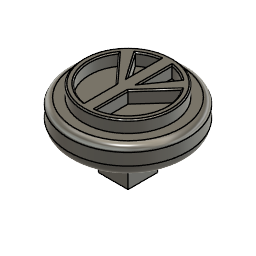
PIN2 (Autodesk Fusion 360 design; units mm, degrees)
Autodesk Fusion 360 part; units mm, degrees
sketch "Sketch2" plane through (0, 6, 0) normal (0, 1, 0) x (-1, 0, 0)
  line L0 (0, -10) -> (0, 0)
  line L1 (0, 0) -> (-5, 0)
  line L2 (-5, 0) -> (-5, -10)
  line L3 (-5, -10) -> (0, -10)
  line L4 (-5, -7.5) -> (0, -7.5)
  line L5 (0, -7.5) -> (0, -2.5)
  line L6 (0, -2.5) -> (-5, -2.5)
  line L7 (-5, -2.5) -> (-5, -7.5)
  dimension "d39" = 5
  dimension "d40" = 5
  dimension "d41" = 2.5
  constraint horizontal L4
  constraint vertical L5
  constraint horizontal L6
  constraint vertical L7
  constraint collinear L2 L7
  measures "d39" distance of L4.start L4.end
  measures "d40" distance of L4.start L6.end
  measures "d41" distance of L3 L4
extrude "Extrude2" add sketch "Sketch2" along normal blind 6 contours L0 L2 L4 L5 L6 L7 makes body 1
sketch "Sketch3" plane through (0, 12, 0) normal (0, 1, 0) x (-1, 0, 0)
  circle A0 centre (-2.5, -5) radius 10
  line L0 (-5, -2.5) -> (-5, -7.5)
  line L1 (-5, -7.5) -> (0, -7.5)
  line L2 (0, -7.5) -> (0, -2.5)
  line L3 (0, -2.5) -> (-5, -2.5)
  dimension "d12" = 20
  measures "d12" diameter of A0
extrude "Extrude3" add sketch "Sketch3" along normal blind 5 contours A0 | L0 L1 L2 L3 makes body 2
fillet "Fillet1" radius 1 1 edges at (11.8233, 17, -8.6162) on bodies 2
fillet "Fillet2" radius 2 1 edges at (11.8233, 12, -8.6162) on bodies 2
sketch "Sketch4" plane through (0, 17, 0) normal (0, 1, 0) x (-1, 0, 0)
  circle A0 centre (-2.5, -5) radius 9
  circle A1 centre (-2.5, -5) radius 6.5
  circle A2 centre (-2.5, -5) radius 7.5
  line L0 (-3.5, -11.4226) -> (-3.5, 1.4226)
  line L1 (-1.5, -11.4226) -> (-1.5, 1.4226)
  line L2 (-1.5, -4) -> (2.8204, -8.7341)
  line L3 (1.4333, -10.1749) -> (-1.5, -6)
  line L4 (-2.5, 1.5) -> (-2.5, -11.5)
  line L5 (-3.5, -4) -> (-7.8204, -8.7341)
  line L6 (-6.4333, -10.1749) -> (-3.5, -6)
  point P0 (-1.5, -11.4226)
  point P1 (-3.5, -11.4226)
  point P2 (-2.5, -11.5)
  point P3 (-1.5, -5)
  point P4 (2.1847, -9.506)
  dimension "d21" = 13
  dimension "d22" = 15
  dimension "d23" = 2
  dimension "d24" = 1
  dimension "d25" = 2
  dimension "d27" = 1
  dimension "d28" = 1
  dimension "d29" = 2
  constraint concentric A0 A1
  constraint concentric A1 A2
  constraint coincident A1 P0
  constraint coincident A1 P1
  constraint coincident A1 P2
  constraint vertical A0.centre L4.end
  constraint coincident P1 L0.start
  constraint coincident A1 L0.end
  constraint vertical L0
  constraint coincident P0 L1.start
  constraint coincident A1 L1.end
  constraint parallel L0 L1
  constraint coincident L1 L2.start
  constraint coincident A1 L2.end
  constraint coincident A1 L3.start
  constraint coincident L1 L3.end
  constraint midpoint L1 P3
  constraint coincident A1 P4
  constraint coincident A1 L4.start
  constraint coincident P2 L4.end
  constraint vertical L4
  constraint symmetric L2.start L4 L5.start
  constraint symmetric L2.end L4 L5.end
  constraint symmetric L3.start L4 L6.start
  constraint symmetric L3.end L4 L6.end
  measures "d21" diameter of A1
  measures "d22" diameter of A2
  measures "d23" distance of P0 P1
  measures "d24" horizontal distance of P0 P2
  measures "d25" distance of L2.end L3.start
  measures "d27" distance of L2.start P3
  measures "d28" distance of L2.end P4
  measures "d29" distance of L2.start L3.end
extrude "Extrude4" add sketch "Sketch4" along normal blind 2 contours A1 L1 L4 | A1 L1 L2 L3 | A1 L0 L4 | A1 L0 L5 L6 | A2 bodies 2
fillet "Fillet3" radius 0.2 13 edges at (4.9666, 19, -8.0874) (5.0443, 19, -10.9813) (3.5, 19, -8.7113) (9.4925, 19, -7.7121) (5.6602, 19, -6.367) (8.4813, 19, -2.4557) (3.5, 19, -1.2887) (1.5, 19, -1.2887) (-3.4813, 19, -2.4557) (-0.6602, 19, -6.367) (0.0334, 19, -8.0874) (-0.0443, 19, -10.9813) (1.5, 19, -8.7113) on bodies 2
